Autodesk Inventor part; units mm, degrees
note: some values were not read from the file. Chosen so that the rebuilt part matches the saved one: sketch regions of "Extrusion30".
(part 2 of 2)
sketch "Sketch70" plane through (0, 1.5, 0) normal (0, 1, 0) x (1, 0, 0)
  line L0 (3.3922, -22.4) -> (-3.6078, -22.4) projected
  line L1 (6.4642, -22.4) -> (6.4642, -4.9) projected
  line L2 (6.4642, -4.9) -> (13.4642, -4.9) projected
  line L3 (13.4642, -4.9) -> (13.4642, -22.4) projected
  line L4 (13.4642, -22.4) -> (6.4642, -22.4) projected
  line L5 (-17.5932, -23.9) -> (-17.5932, -11.7729) projected
  line L6 (3.3922, -22.4) -> (3.3922, -22.9)
  line L7 (3.3922, -22.9) -> (-3.6078, -22.9)
  line L8 (-3.6078, -22.9) -> (-3.6078, -22.4)
  line L9 (-3.6078, -22.4) -> (3.3922, -22.4)
  line L10 (3.3922, -22.9) -> (-3.6078, -22.9)
  line L11 (-3.6078, -22.9) -> (-3.6078, -4.9)
  line L12 (-3.6078, -4.9) -> (3.3922, -4.9)
  line L13 (3.3922, -4.9) -> (3.3922, -22.9)
  line L14 (13.4642, -22.9) -> (6.4642, -22.9)
  line L15 (6.4642, -22.9) -> (6.4642, -4.9)
  line L16 (6.4642, -4.9) -> (13.4642, -4.9)
  line L17 (13.4642, -4.9) -> (13.4642, -22.9)
  point P0 (0, 0)
  dimension "d343" = 0.5
  dimension "d344" = 7
  dimension "d345" = 18
  dimension "d346" = 7
  constraints: 24 end point, 6 parallel, 3 perpendicular, 2 horizontal, 1 collinear
  measures "d343" distance of L0.start L6.end
  measures "d344" distance of L11.end L12.end
  measures "d345" distance of L10.end L11.end
  measures "d346" distance of L1.end L16.end
extrude "Extrusion65" cut sketch "Sketch70" against normal blind 1.5 contours L6 L7 L8 L0 | L4 L17 L14 L15
sketch "Sketch71" plane through (0, 1.5, 0) normal (0, 1, 0) x (1, 0, 0)
  line L0 (6.4642, -4.9) -> (13.4642, -4.9) projected
  line L1 (-3.6078, -4.9) -> (3.3922, -4.9) projected
  line L2 (-3.6078, -3.9) -> (3.3922, -3.9)
  line L3 (6.4642, -3.9) -> (13.4642, -3.9)
  line L4 (-3.4042, -4.9) -> (3.3922, -4.9)
  line L5 (13.4642, -4.9) -> (6.4642, -4.9)
  line L6 (6.4642, -4.9) -> (6.4642, -3.9)
  line L7 (13.4642, -4.9) -> (13.4642, -3.9)
  line L8 (6.4642, -4.9) -> (6.4642, -3.9)
  line L9 (13.4642, -4.9) -> (6.4642, -4.9)
  line L10 (3.3922, -3.9) -> (3.3922, -4.9)
  line L11 (3.3922, -4.9) -> (-3.6078, -4.9)
  line L12 (-3.6078, -4.9) -> (-3.6078, -3.9)
  point P0 (3.3922, -22.9)
  point P1 (0, 0)
  dimension "d349" = 7
  dimension "d351" = 7
  constraints: 22 end point, 4 collinear, 1 point on line
  measures "d349" distance of L2.start L2.end
  measures "d351" distance of L3.start L3.end
extrude "Extrusion66" cut sketch "Sketch71" against normal blind 1.5
sketch "Sketch75" plane through (0, 1.5, 0) normal (0, 1, 0) x (1, 0, 0)
  line L0 (-14, 20) -> (14, 20) projected
  line L1 (-14, 20) -> (0, 20)
  line L2 (0, 20) -> (0, 11.7)
  line L3 (0, 11.7) -> (-11.6, 11.7)
  line L4 (-11.6, 11.7) -> (12, 11.7)
  line L5 (12, 11.7) -> (12, -0.7)
  line L6 (12, -0.7) -> (-11.6, -0.7)
  line L7 (-11.6, -0.7) -> (-11.6, 11.7)
  point P0 (0, 0)
  dimension "d359" = 8.3
  dimension "d360" = 11.6
  dimension "d361" = 23.6
  dimension "d362" = 12.4
  constraints: 14 end point, 3 perpendicular, 2 parallel, 1 horizontal, 1 midpoint
  measures "d359" distance of L1.end L2.end
  measures "d360" distance of L2.end L3.end
  measures "d361" distance of L5.end L6.end
  measures "d362" distance of L4.end L5.end
extrude "Extrusion67" cut sketch "Sketch75" against normal blind 1.5
sketch "Sketch76" plane through (0, 1.5, 0) normal (0, 1, 0) x (1, 0, 0)
  line L0 (-11.6, -0.7) -> (-11.6, 11.7) projected
  circle A0 centre (13.95, 5.5) radius 1.5 projected
  circle A1 centre (-13.95, 5.5) radius 1.5 projected
  line L1 (6.4642, -3.9) -> (13.4642, -3.9) projected
  line L2 (-13.95, 5.5) -> (13.95, 5.5)
  line L3 (-11.6, 11.7) -> (-12, 11.7)
  line L4 (-12, 11.7) -> (-12, -0.7)
  line L5 (-12, -0.7) -> (-11.6, -0.7)
  line L6 (-11.6, 11.7) -> (-11.6, -0.7)
  point P0 (0, 0)
  dimension "d365" = 27.9
  dimension "d366" = 0.4
  constraints: 10 end point, 3 parallel, 2 perpendicular
  measures "d365" distance of L2.start L2.end
  measures "d366" distance of L0.end L3.end
extrude "Extrusion68" cut sketch "Sketch76" against normal blind 1.5 contours L5 L4 L2 L0 | L2 L4 L3 L0
sketch "Sketch77" plane through (0, 1.5, 0) normal (0, 1, 0) x (1, 0, 0)
  line L0 (-12, 11.7) -> (12, 11.7) projected
  line L1 (12, -0.7) -> (-12, -0.7) projected
  line L2 (-12, -0.7) -> (-12, 11.7) projected
  line L3 (-12, 11.7) -> (-12, -0.7)
  line L4 (-12, -0.7) -> (-11.7, -0.7)
  line L5 (-11.7, -0.7) -> (-11.7, 11.7)
  line L6 (-12, 11.7) -> (-11.7, 11.7)
  line L7 (12, 11.7) -> (12, -0.7)
  line L8 (12, -0.7) -> (11.7, -0.7)
  line L9 (11.7, -0.7) -> (11.7, 11.7)
  line L10 (11.7, 11.7) -> (12, 11.7)
  point P0 (0, 0)
  dimension "d370" = 0.3
  dimension "d371" = 0.3
  constraints: 16 end point, 5 perpendicular, 4 point on line, 1 collinear
  measures "d370" distance of L1.end L4.end
  measures "d371" distance of L1.start L8.end
extrude "Extrusion69" add sketch "Sketch77" against normal blind 1.5 contours L0 L5 L1 L2 | L0 L7 L1 L9
sketch "Sketch78" plane through (-17.5932, 0, 25.4) normal (0, 0, 1) x (1, 0, 0)
  line L0 (0, 11.5) -> (35.1864, 11.5) projected
  line L1 (17.5932, 11.5) -> (17.5932, 6.5)
  circle A0 centre (17.5932, 6.5) radius 2.5
  point P0 (17.5932, 0)
  dimension "d374" = 5
  dimension "d375" = 5
  constraints: 2 end point, 1 centre point, 1 coincident, 1 midpoint, 1 perpendicular
  measures "d374" distance of L1.start L1.end
  measures "d375" diameter of A0
extrude "Extrusion70" cut sketch "Sketch78" against normal blind 1.5
sketch "Sketch79" plane through (-17.5932, 0, 25.4) normal (0, 0, 1) x (1, 0, 0)
  circle A0 centre (17.5932, 6.5) radius 2.5 projected
  line L0 (0, 11.5) -> (35.1864, 11.5) projected
  line L1 (17.5932, 6.5) -> (11.2932, 6.5)
  line L2 (11.2932, 6.5) -> (23.8932, 6.5)
  circle A1 centre (11.2932, 6.5) radius 1.5
  circle A2 centre (23.8932, 6.5) radius 1.5
  point P0 (17.5932, 0)
  dimension "d378" = 6.3
  dimension "d379" = 12.6
  dimension "d380" = 3
  dimension "d381" = 3
  constraints: 4 end point, 2 centre point, 2 coincident, 1 collinear, 1 parallel
  measures "d378" distance of L1.start L1.end
  measures "d379" distance of L1.end L2.end
  measures "d380" diameter of A1
  measures "d381" diameter of A2
extrude "Extrusion71" cut sketch "Sketch79" against normal blind 1.5 contours A1 | A2
sketch "Sketch82" plane through (0, 0, 0) normal (0, -1, 0) x (1, 0, 0)
  line L0 (-3.6078, 3.9) -> (-3.6078, 22.9) projected
  line L1 (-3.6078, 22.9) -> (3.3922, 22.9) projected
  line L2 (3.3922, 22.9) -> (3.3922, 3.9) projected
  line L3 (3.3922, 3.9) -> (-3.6078, 3.9) projected
  line L4 (13.4642, 22.9) -> (13.4642, 3.9) projected
  line L5 (13.4642, 3.9) -> (6.4642, 3.9) projected
  line L6 (6.4642, 3.9) -> (6.4642, 22.9) projected
  line L7 (6.4642, 22.9) -> (13.4642, 22.9) projected
  point P0 (0, 0)
extrude "Extrusion72" add sketch "Sketch82" against normal blind 1.5
sketch "Sketch83" plane through (0, 0, 0) normal (0, -1, 0) x (1, 0, 0)
  line L0 (-14.0932, 3.9) -> (-7.0932, 3.9)
  line L1 (-7.0932, 3.9) -> (-7.0932, 22.9)
  line L2 (-7.0932, 22.9) -> (-14.0932, 22.9)
  line L3 (-14.0932, 22.9) -> (-14.0932, 3.9)
  line L4 (14.0932, 3.9) -> (7.0932, 3.9)
  line L5 (7.0932, 3.9) -> (7.0932, 22.9)
  line L6 (14.0932, 22.9) -> (7.0932, 22.9)
  line L7 (7.0932, 22.9) -> (14.0932, 22.9)
  line L8 (14.0932, 22.9) -> (14.0932, 3.9)
  point P0 (0, 0)
  dimension "d395" = 7
  dimension "d396" = 19
  dimension "d399" = 7
  constraints: 18 end point, 1 collinear
  measures "d395" distance of L0.start L0.end
  measures "d396" distance of L0.end L1.end
  measures "d399" distance of L4.start L4.end
extrude "Extrusion73" cut sketch "Sketch83" against normal blind 1.5
sketch "Sketch85" plane through (0, 0, 0) normal (0, -1, 0) x (1, 0, 0)
  line L0 (-7.0932, 22.9) -> (-7.0932, 3.9) projected
  line L1 (-7.0932, 3.9) -> (-14.0932, 3.9) projected
  line L2 (-14.0932, 3.9) -> (-14.0932, 22.9) projected
  line L3 (-14.0932, 22.9) -> (-7.0932, 22.9) projected
  line L4 (7.0932, 22.9) -> (14.0932, 22.9) projected
  line L5 (14.0932, 22.9) -> (14.0932, 3.9) projected
  line L6 (14.0932, 3.9) -> (7.0932, 3.9) projected
  line L7 (7.0932, 3.9) -> (7.0932, 22.9) projected
  point P0 (0, 0)
extrude "Extrusion74" add sketch "Sketch85" against normal blind 1.5
sketch "Sketch86" plane through (0, 0, 0) normal (0, -1, 0) x (1, 0, 0)
  line L0 (17.5932, 25.4) -> (-17.5932, 25.4) projected
  line L1 (11.7, 0.7) -> (11.7, -11.7) projected
  line L2 (0, 25.4) -> (0, 3.9)
  line L3 (0, 3.9) -> (0, 5.4)
  circle A0 centre (0, 5.4) radius 1.5
  line L4 (0, 5.4) -> (0, 24.4)
  line L5 (0, 24.4) -> (0, 22.9)
  circle A1 centre (0, 22.9) radius 1.5
  line L6 (-1.5, 22.9) -> (-1.5, 5.4)
  line L7 (1.5, 22.9) -> (1.5, 5.4)
  point P0 (0, 0)
  dimension "d406" = 1.5
  dimension "d407" = 3
  dimension "d409" = 1.5
  dimension "d410" = 3
  constraints: 12 end point, 4 point on circle, 4 tangent, 3 point on line, 2 centre point, 2 coincident, 1 midpoint, 1 parallel
  measures "d406" distance of L2.end L3.end
  measures "d407" diameter of A0
  measures "d409" distance of L4.end L5.end
  measures "d410" diameter of A1
extrude "Extrusion75" cut sketch "Sketch86" against normal blind 1.5
sketch "Sketch87" plane through (0, 0, 0) normal (0, -1, 0) x (1, 0, 0)
  line L0 (-1.5, 5.4) -> (-1.5, 22.9) projected
  arc A0 (1.5, 22.9) -> (-1.5, 22.9) centre (0, 22.9) ccw projected
  line L1 (1.5, 22.9) -> (1.5, 5.4) projected
  arc A1 (-1.5, 5.4) -> (1.5, 5.4) centre (0, 5.4) ccw projected
  line L2 (11.7, 0.7) -> (11.7, -11.7) projected
  line L3 (0, 22.9) -> (0, 8.4)
  circle A2 centre (0, 8.4) radius 1.5
  circle A3 centre (0, 5.4) radius 1.5
  line L4 (-1.5, 5.4) -> (-1.5, 8.4)
  line L5 (1.5, 8.4) -> (1.5, 5.4)
  point P0 (0, 0)
  dimension "d413" = 14.5
  dimension "d414" = 3
  constraints: 6 end point, 3 point on line, 2 coincident, 2 point on circle, 1 centre point, 1 horizontal alignment, 1 parallel, 2 other
  measures "d413" distance of L3.start L3.end
  measures "d414" diameter of A2
extrude "Extrusion76" add sketch "Sketch87" against normal blind 1.5 contours A3 A1 | L0 A2 A3 | A3 A2 L1
sketch "Sketch88" plane through (0, 0, 0) normal (0, -1, 0) x (1, 0, 0)
  line L0 (-1.5, 8.4) -> (-1.5, 22.9) projected
  arc A0 (1.5, 22.9) -> (-1.5, 22.9) centre (0, 22.9) ccw projected
  line L1 (1.5, 22.9) -> (1.5, 8.4) projected
  arc A1 (-1.5, 8.4) -> (1.5, 8.4) centre (0, 8.4) ccw projected
  line L2 (17.5932, 25.4) -> (-17.5932, 25.4) projected
  line L3 (11.7, 0.7) -> (11.7, -11.7) projected
  line L4 (0, 25.4) -> (0, 22.4)
  circle A2 centre (0, 22.9) radius 1.5
  line L5 (0, 22.4) -> (0, 20.9)
  circle A3 centre (0, 20.9) radius 1.5
  line L6 (0, 8.4) -> (0, 10.4)
  circle A4 centre (0, 10.4) radius 1.5
  circle A5 centre (0, 8.4) radius 1.5
  line L7 (-1.5, 8.4) -> (-1.5, 10.4)
  line L8 (1.5, 10.4) -> (1.5, 8.4)
  line L9 (1.5, 22.9) -> (1.5, 20.9)
  line L10 (-1.4949, 23.0232) -> (-1.5, 20.9)
  point P0 (0, 0)
  dimension "d417" = 3
  dimension "d418" = 1.5
  dimension "d419" = 3
  dimension "d420" = 2
  dimension "d421" = 3
  dimension "d422" = 3
  constraints: 14 end point, 5 point on circle, 4 coincident, 4 point on line, 3 centre point, 2 parallel, 1 collinear, 1 midpoint, 1 tangent, 3 other
  measures "d417" distance of L4.start L4.end
  measures "d418" distance of L4.end L5.end
  measures "d419" diameter of A3
  measures "d420" distance of L6.start L6.end
  measures "d421" diameter of A4
  measures "d422" diameter of A5
extrude "Extrusion77" add sketch "Sketch88" against normal blind 1.5 contours A5 A4 A1 | L0 A4 A5 | A5 A4 L1
sketch "Sketch89" plane through (0, 0, 0) normal (0, -1, 0) x (1, 0, 0)
  line L0 (-1.5, 10.4) -> (-1.5, 22.9) projected
  arc A0 (1.5, 22.9) -> (-1.5, 22.9) centre (0, 22.9) ccw projected
  line L1 (1.5, 22.9) -> (1.5, 10.4) projected
  line L2 (11.7, 0.7) -> (11.7, -11.7) projected
  line L3 (0, 22.9) -> (0, 21.4)
  circle A1 centre (0, 21.4) radius 1.5
  circle A2 centre (0, 22.9) radius 1.5
  line L4 (-1.5, 22.9) -> (-1.5, 21.4)
  line L5 (1.5, 22.9) -> (1.5, 21.4)
  point P0 (0, 0)
  dimension "d425" = 1.5
  constraints: 6 end point, 3 point on circle, 2 centre point, 2 coincident, 2 point on line, 1 parallel
  measures "d425" distance of L3.start L3.end
extrude "Extrusion78" add sketch "Sketch89" against normal blind 1.5 contours L0 A2 A1 | A0 A2 A1 | A1 A2 L1
sketch "Sketch90" plane through (0, 0, 0) normal (0, -1, 0) x (1, 0, 0)
  arc A0 (-1.5, 10.4) -> (1.5, 10.4) centre (0, 10.4) ccw projected
  line L0 (11.7, 0.7) -> (11.7, -11.7) projected
  line L1 (0, 8.9) -> (0, 7.4)
  circle A1 centre (0, 7.4) radius 1.5
  line L2 (-1.5, 10.4) -> (-1.5, 7.4)
  line L3 (1.5, 10.4) -> (1.5, 7.4)
  circle A2 centre (0, 10.4) radius 1.5
  point P0 (0, 0)
  dimension "d428" = 1.5
  constraints: 6 end point, 6 point on circle, 2 coincident, 2 parallel, 2 tangent, 1 centre point, 1 vertical alignment, 2 other
  measures "d428" distance of L1.start L1.end
extrude "Extrusion79" cut sketch "Sketch90" against normal blind 1.5 contours A0 A1 L2 | A0 L3 A1 | A1
sketch "Sketch91" plane through (0, 0, 0) normal (0, -1, 0) x (1, 0, 0)
  line L0 (-1.5, 7.4) -> (-1.5, 21.4) projected
  arc A0 (1.5, 21.4) -> (-1.5, 21.4) centre (0, 21.4) ccw projected
  line L1 (1.5, 21.4) -> (1.5, 7.4) projected
  arc A1 (-1.5, 7.4) -> (1.5, 7.4) centre (0, 7.4) ccw projected
  point P0 (0, 0)
extrude "Extrusion80" add sketch "Sketch91" against normal blind 1.5
sketch "Sketch92" plane through (0, 0, 0) normal (0, -1, 0) x (1, 0, 0)
  line L0 (17.5932, 25.4) -> (-17.5932, 25.4) projected
  line L1 (-11.7, 0.7) -> (11.7, 0.7) projected
  line L2 (11.7, 0.7) -> (11.7, -11.7) projected
  line L3 (0, 0.7) -> (0, 3.7)
  circle A0 centre (0, 3.7) radius 1.5
  line L4 (0, 25.4) -> (0, 22.4)
  circle A1 centre (0, 22.4) radius 1.5
  point P0 (0, 0)
  dimension "d433" = 3
  dimension "d434" = 3
  dimension "d435" = 3
  dimension "d436" = 3
  constraints: 4 end point, 2 centre point, 2 coincident, 2 midpoint, 1 collinear, 1 parallel
  measures "d433" distance of L3.start L3.end
  measures "d434" diameter of A0
  measures "d435" distance of L4.start L4.end
  measures "d436" diameter of A1
extrude "Extrusion81" cut sketch "Sketch92" against normal blind 1.5
sketch "Sketch93" plane through (0, 0, 0) normal (0, -1, 0) x (1, 0, 0)
  circle A0 centre (0, 22.4) radius 1.5 projected
  point P0 (0, 0)
extrude "Extrusion82" add sketch "Sketch93" against normal blind 1.5
sketch "Sketch94" plane through (0, 1.5, 0) normal (0, 1, 0) x (1, 0, 0)
  line L0 (-17.5932, -23.9) -> (17.5932, -23.9) projected
  line L1 (-11.7, -0.7) -> (-11.7, 11.7) projected
  line L2 (0, -23.9) -> (0, -20.9)
  circle A0 centre (0, -20.9) radius 1.5
  point P0 (0, 0)
  dimension "d441" = 3
  dimension "d442" = 3
  constraints: 2 end point, 1 centre point, 1 coincident, 1 midpoint, 1 parallel
  measures "d441" distance of L2.start L2.end
  measures "d442" diameter of A0
extrude "Extrusion83" cut sketch "Sketch94" against normal blind 1.5
sketch "Sketch96" plane through (0, 0, 0) normal (0, -1, 0) x (1, 0, 0)
  circle A0 centre (0, 20.9) radius 1.5 projected
  circle A1 centre (0, 3.7) radius 1.5 projected
  line L0 (17.5932, 11.7729) -> (17.5932, 25.4) projected
  line L1 (17.5932, 25.4) -> (-17.5932, 25.4) projected
  line L2 (-17.5932, 25.4) -> (-17.5932, 11.7729) projected
  arc A2 (-26, -4) -> (-17.5932, 11.7729) centre (-36.5932, 11.7729) ccw projected
  line L3 (-26, -4) -> (-14, -20) projected
  line L4 (-14, -20) -> (14, -20) projected
  line L5 (14, -20) -> (26, -4) projected
  arc A3 (17.5932, 11.7729) -> (26, -4) centre (36.5932, 11.7729) ccw projected
  circle A4 centre (-13.95, -5.5) radius 1.5 projected
  circle A5 centre (13.95, -5.5) radius 1.5 projected
  circle A6 centre (12.72, -16.04) radius 1.5 projected
  circle A7 centre (21.72, -4.04) radius 1.5 projected
  circle A8 centre (-21.72, -4.04) radius 1.5 projected
  circle A9 centre (-12.72, -16.04) radius 1.5 projected
  line L6 (11.7, -11.7) -> (-11.7, -11.7) projected
  line L7 (-11.7, -11.7) -> (-11.7, 0.7) projected
  line L8 (-11.7, 0.7) -> (11.7, 0.7) projected
  line L9 (11.7, 0.7) -> (11.7, -11.7) projected
  point P0 (0, 0)
extrude "Extrusion84" add sketch "Sketch96" along normal blind 0.5
sketch "Sketch97" plane through (-17.5932, 11.5, 25.4) normal (0, 0, 1) x (1, 0, 0)
  circle A0 centre (11.2932, -5) radius 1.5 projected
  circle A1 centre (23.8932, -5) radius 1.5 projected
  circle A2 centre (17.5932, -5) radius 2.5 projected
  line L0 (0, -12) -> (0, 0) projected
  line L1 (35.1864, -12) -> (0, -12) projected
  line L2 (35.1864, -12) -> (35.1864, 0) projected
  line L3 (0, 0) -> (35.1864, 0) projected
  point P0 (17.5932, -11.5)
extrude "Extrusion85" add sketch "Sketch97" along normal blind 0.5
sketch "Sketch98" plane through (-17.5932, 11.5, 25.9) normal (0, 0, 1) x (1, 0, 0)
  line L0 (0, 0) -> (0, -12) projected
  line L1 (35.1864, -12) -> (35.1864, 0) projected
  line L2 (35.1864, 0) -> (0, 0) projected
  line L3 (35.1864, -5) -> (30.1864, -5)
  line L4 (0, -5) -> (5, -5)
  circle A0 centre (5, -5) radius 1.5
  circle A1 centre (30.1864, -5) radius 1.5
  point P0 (17.5932, -11.5)
  dimension "d449" = 5
  dimension "d450" = 5
  dimension "d451" = 3
  dimension "d452" = 3
  constraints: 4 end point, 2 centre point, 2 coincident, 2 point on line, 1 collinear, 1 parallel
  measures "d449" distance of L3.start L3.end
  measures "d450" distance of L4.start L4.end
  measures "d451" diameter of A0
  measures "d452" diameter of A1
extrude "Extrusion86" cut sketch "Sketch98" against normal blind 2
sketch "Sketch99" plane through (-17.5932, 11.5, 25.9) normal (0, 0, 1) x (1, 0, 0)
  circle A0 centre (23.8932, -5) radius 1.5 projected
  circle A1 centre (11.2932, -5) radius 1.5 projected
  circle A2 centre (11.2932, -5) radius 1
  circle A3 centre (23.8932, -5) radius 1
  point P0 (17.5932, -11.5)
  dimension "d455" = 2
  dimension "d456" = 2
  constraints: 2 centre point, 2 coincident
  measures "d455" diameter of A2
  measures "d456" diameter of A3
extrude "Extrusion87" add sketch "Sketch99" against normal blind 2
sketch "Sketch101" plane through (-17.5932, 11.5, 25.9) normal (0, 0, 1) x (1, 0, 0)
  circle A0 centre (23.8932, -5) radius 1 projected
  circle A1 centre (11.2932, -5) radius 1 projected
  point P0 (17.5932, -11.5)
extrude "Extrusion88" add sketch "Sketch101" against normal blind 2
sketch "Sketch102" plane through (-17.5932, 11.5, 25.9) normal (0, 0, 1) x (1, 0, 0)
  circle A0 centre (5, -5) radius 1.5 projected
  circle A1 centre (30.1864, -5) radius 1.5 projected
  point P0 (17.5932, -11.5)
extrude "Extrusion89" add sketch "Sketch102" against normal blind 2
sketch "Sketch103" plane through (-17.5932, 11.5, 25.9) normal (0, 0, 1) x (1, 0, 0)
  circle A0 centre (5.0002, -5) radius 1.5
  circle A1 centre (30.1862, -5) radius 1.5
  point P0 (17.5932, -11.5)
  dimension "d464" = 3
  dimension "d465" = 3
  constraints: 2 centre point
  measures "d464" diameter of A0
  measures "d465" diameter of A1
extrude "Extrusion90" cut sketch "Sketch103" against normal blind 2
body "Solid1"
